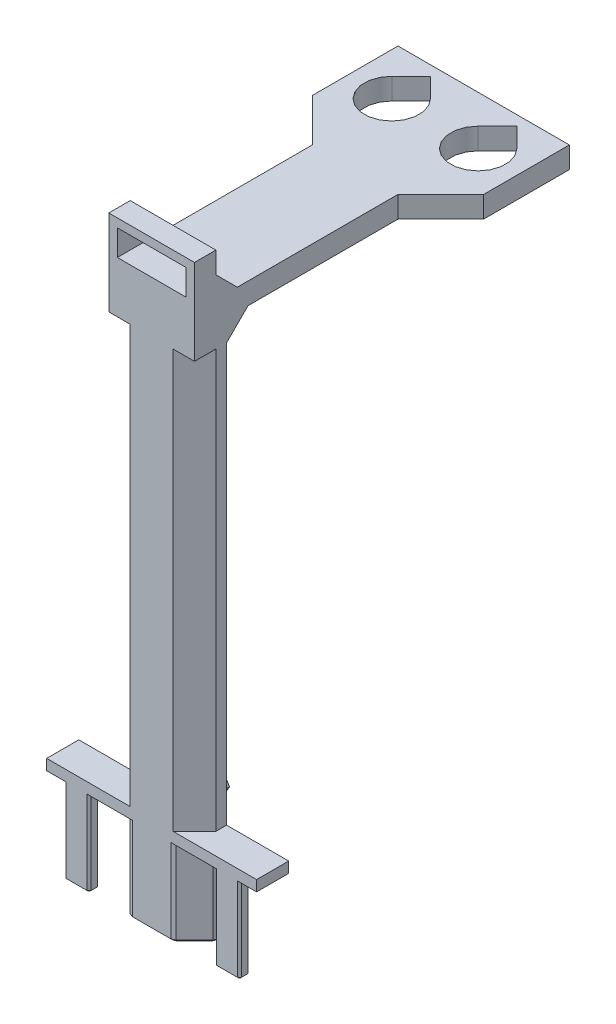
# Autodesk Inventor part: Vertical Beam Prototype
Saved by Autodesk Inventor 2022 (Build 260153000, 153)
## iProperties
Created: 2021-05-30
Part Number: Vertical Beam Prototype
Material: Generic
Document SubType Name: Modeling
Designer: sidsa
Density: 1 g/cm^3
Appearance: Silver
Author: sidsa
## iProperties of the stored document Vertical Beam Prototype_3DPrint.ipt
Created: 2021-05-30
Part Number: Vertical Beam Prototype_3DPrint
Material: Generic
Document SubType Name: Modeling
Designer: sidsa
Density: 1 g/cm^3
Appearance: Default
Author: sidsa
Autodesk Inventor part; units mm, degrees
ref_plane "YZ Plane" through (0, 0, 0) normal (1, 0, 0) x (0, 1, 0)
ref_plane "XZ Plane" through (0, 0, 0) normal (0, 1, 0) x (-1, 0, 0)
ref_plane "XY Plane" through (0, 0, 0) normal (0, 0, 1) x (1, 0, 0)
sketch "Sketch1" plane through (0, 0, 0) normal (0, 0, 1) x (1, 0, 0)
  line L0 (0, 0) -> (25.4, 0)
  line L1 (25.4, 0) -> (25.4, 165.1)
  line L2 (25.4, 165.1) -> (0, 165.1)
  line L3 (0, 165.1) -> (0, 0)
  line L4 (16.2837, 38.7604) -> (19.9133, 32.4739)
  line L5 (19.9133, 32.4739) -> (16.2837, 26.1874)
  line L6 (16.2837, 26.1874) -> (9.0247, 26.1874)
  line L7 (9.0247, 26.1874) -> (5.3952, 32.4739)
  line L8 (5.3952, 32.4739) -> (9.0247, 38.7604)
  line L9 (9.0247, 38.7604) -> (16.2837, 38.7604)
  line L10 (12.7, 0) -> (12.6542, 32.4739)
  dimension "d0" = 25.4
  dimension "d1" = 165.1
  dimension "d2" = 12.573
  dimension "d3" = 26.1874
  constraints: 22 end point, 3 parallel, 1 horizontal, 1 midpoint, 1 perpendicular, 13 other
  measures "d0" distance of L1.end L2.end
  measures "d1" distance of L0.end L1.end
  measures "d2" distance between parallel lines of L6 L9
  measures "d3" distance between parallel lines of L0 L6
extrude "Extrusion1" add sketch "Sketch1" along normal blind 3.175
sketch "Sketch2" plane through (0, 0, 0) normal (0, 0, -1) x (-1, 0, 0)
  line L0 (-25.4, 0) -> (-25.4, 165.1) projected
  line L1 (0, 0) -> (-25.4, 0) projected
  line L2 (0, 165.1) -> (0, 0) projected
  line L3 (-25.4, 165.1) -> (0, 165.1) projected
  line L4 (-16.2837, 26.1874) -> (-9.0247, 26.1874) projected
  line L5 (-19.9133, 32.4739) -> (-16.2837, 26.1874) projected
  line L6 (-16.2837, 38.7604) -> (-19.9133, 32.4739) projected
  line L7 (-9.0247, 38.7604) -> (-16.2837, 38.7604) projected
  line L8 (-5.3952, 32.4739) -> (-9.0247, 38.7604) projected
  line L9 (-9.0247, 26.1874) -> (-5.3952, 32.4739) projected
  line L10 (-16.2984, 26.1967) -> (-19.9179, 32.4658) projected
  line L11 (-5.4399, 32.4658) -> (-9.0594, 26.1967) projected
  line L12 (-9.0594, 26.1967) -> (-16.2984, 26.1967) projected
  line L13 (-16.2984, 26.1967) -> (-19.9179, 32.4658) projected
  line L14 (-19.9179, 32.4658) -> (-16.2984, 38.735) projected
  line L15 (-16.2984, 38.735) -> (-9.0594, 38.735) projected
  line L16 (-9.0594, 38.735) -> (-5.4399, 32.4658) projected
  line L17 (-41.2539, 1.27) -> (-34.9039, 1.27) projected
  line L18 (15.8961, 1.27) -> (15.8961, 63.5) projected
  line L19 (-41.2539, 63.5) -> (15.8961, 63.5) projected
  line L20 (-41.2539, 1.27) -> (-41.2539, 63.5) projected
  line L21 (6.3711, 1.27) -> (6.3711, 26.67) projected
  line L22 (6.3711, 26.67) -> (9.5461, 26.67) projected
  line L23 (9.5461, 26.67) -> (9.5461, 1.27) projected
  line L24 (9.5461, 1.27) -> (15.8961, 1.27) projected
  line L25 (-34.9039, 1.27) -> (-34.9039, 26.67) projected
  line L26 (-34.9039, 26.67) -> (-31.7289, 26.67) projected
  line L27 (-31.7289, 26.67) -> (-31.7289, 1.27) projected
  line L28 (-31.7289, 1.27) -> (6.3711, 1.27) projected
  dimension "d32" = 12.573
  dimension "d33" = 12.5383
  measures "d32" distance between parallel lines of L7 L4
  measures "d33" distance between parallel lines of L12 L15
extrude "Extrusion2" add sketch "Sketch2" along normal blind 6.35 and the other way blind 3.175 contours L5 L12 L11 L16 L15 L6 L7 L8 L9 L4 | L5 L6 L15 L16 L11 L12
sketch "Sketch3" plane through (0, 0, 3.175) normal (0, 0, 1) x (1, 0, 0)
  line L0 (25.4, 0) -> (25.4, 165.1) projected
  line L1 (25.4, 165.1) -> (0, 165.1) projected
  line L2 (0, 165.1) -> (0, 0) projected
  line L3 (0, 0) -> (25.4, 0) projected
extrude "Extrusion3" add sketch "Sketch3" along normal blind 6.35
chamfer "Chamfer1" distance 6.35 angle 45 2 edges at (25.4, 82.55, 9.525) (0, 82.55, 9.525)
sketch "Sketch5" plane through (9.0247, 38.7604, 0) normal (0, 1, 0) x (1, 0, 0)
  line L0 (7.259, 0) -> (7.259, 6.35) projected
  line L1 (32.2292, 2.54) -> (-24.9208, 2.54) projected
  line L2 (0, 0) -> (0, 6.35) projected
  line L3 (7.259, 0) -> (7.259, 6.35) projected
  line L4 (0, 6.35) -> (0, 0) projected
  line L5 (7.259, 2.54) -> (0, 2.54)
  line L6 (0, 2.54) -> (0, 6.35)
  line L7 (0, 6.35) -> (7.259, 6.35)
  line L8 (7.259, 6.35) -> (7.259, 2.54)
  line L9 (5.989, 3.175) -> (1.27, 3.175)
  line L10 (1.27, 3.175) -> (1.27, 5.715)
  line L11 (1.27, 5.715) -> (5.989, 5.715)
  line L12 (5.989, 5.715) -> (5.989, 3.175)
  point P0 (-9.0247, 0)
  dimension "d25" = 0.635
  dimension "d26" = 1.27
  dimension "d27" = 0.635
  dimension "d28" = 1.27
  dimension "d29" = 2.54
  constraints: 16 end point, 4 parallel, 2 horizontal, 2 perpendicular, 2 point on line
  measures "d25" distance between parallel lines of L1 L9
  measures "d26" distance between parallel lines of L2 L10
  measures "d27" distance between parallel lines of L7 L11
  measures "d28" distance between parallel lines of L0 L12
  measures "d29" distance between parallel lines of L11 L9
extrude "Extrusion5" cut sketch "Sketch5" against normal blind 12.7 contours L9 L10 L11 L12
sketch "Sketch6" plane through (0, 0, 0) normal (0, 0, -1) x (-1, 0, 0)
  line L0 (-25.4, 0) -> (-25.4, 165.1) projected
  line L1 (0, 0) -> (-25.4, 0) projected
  line L2 (0, 165.1) -> (0, 0) projected
  line L3 (-25.4, 165.1) -> (0, 165.1) projected
  line L4 (-16.2837, 26.1874) -> (-9.0247, 26.1874) projected
  line L5 (-19.9133, 32.4739) -> (-16.2837, 26.1874) projected
  line L6 (-16.2837, 38.7604) -> (-19.9133, 32.4739) projected
  line L7 (-9.0247, 38.7604) -> (-16.2837, 38.7604) projected
  line L8 (-5.3952, 32.4739) -> (-9.0247, 38.7604) projected
  line L9 (-9.0247, 26.1874) -> (-5.3952, 32.4739) projected
  line L10 (0, 165.1) -> (0, 0) projected
  line L11 (-25.4, 165.1) -> (0, 165.1)
  line L12 (0, 165.1) -> (0, 158.75)
  line L13 (0, 158.75) -> (-25.4, 158.75)
  line L14 (-25.4, 158.75) -> (-25.4, 165.1)
  point P0 (-25.4, 158.75)
  dimension "d34" = 6.35
  constraints: 8 end point, 2 parallel, 1 horizontal, 1 perpendicular, 1 point on line
  measures "d34" distance of L11.end L12.end
extrude "Extrusion6" add sketch "Sketch6" along normal blind 88.9 contours L0 L3 L2 L13
sketch "Sketch7" plane through (0, 0, 3.175) normal (-1, 0, 0) x (0, 0, 1)
  line L0 (-92.075, 165.1) -> (0, 165.1) projected
  line L1 (-3.175, 158.75) -> (-92.075, 158.75) projected
  line L2 (-92.075, 165.1) -> (-66.675, 165.1)
  line L3 (-66.675, 165.1) -> (-66.675, 158.75)
  line L4 (-66.675, 158.75) -> (-92.075, 158.75)
  line L5 (-92.075, 158.75) -> (-92.075, 165.1)
  point P0 (-3.175, 0)
  dimension "d37" = 25.4
  constraints: 8 end point, 2 parallel, 1 horizontal, 1 perpendicular, 1 point on line
  measures "d37" distance of L3.end L4.end
extrude "Extrusion7" add sketch "Sketch7" along normal blind 12.7
sketch "Sketch8" plane through (25.4, 0, 3.175) normal (1, 0, 0) x (0, 0, -1)
  line L0 (92.075, 165.1) -> (0, 165.1) projected
  line L1 (92.075, 165.1) -> (66.675, 165.1)
  line L2 (66.675, 165.1) -> (66.675, 158.75)
  line L3 (66.675, 158.75) -> (92.075, 158.75)
  line L4 (92.075, 158.75) -> (92.075, 165.1)
  point P0 (3.175, 0)
  dimension "d40" = 25.4
  dimension "d41" = 6.35
  constraints: 8 end point, 2 parallel, 1 horizontal, 1 perpendicular
  measures "d40" distance of L3.end L2.end
  measures "d41" distance of L2.end L1.end
extrude "Extrusion8" add sketch "Sketch8" along normal blind 12.7
sketch "Sketch9" plane through (6.35, 165.1, 9.525) normal (0, 1, 0) x (1, 0, 0)
  circle A0 centre (-6.227, 72.0756) radius 6.55 projected
  circle A1 centre (19.373, 72.0756) radius 6.55 projected
  line L0 (31.75, 98.425) -> (31.75, 73.025) projected
  line L1 (-19.05, 73.025) -> (-19.05, 98.425) projected
  line L2 (31.75, 73.025) -> (31.75, 98.425) projected
  line L3 (31.75, 83.986) -> (25.8752, 83.986)
  line L4 (12.8707, 83.986) -> (-19.05, 83.986)
  line L5 (31.75, 83.986) -> (27.2796, 83.986)
  line L6 (27.2796, 83.986) -> (19.1516, 83.986)
  circle A2 centre (19.1516, 83.986) radius 8.128
  line L7 (-19.05, 83.986) -> (-6.4516, 83.986)
  circle A3 centre (-6.4516, 83.986) radius 8.128
  line L8 (5.0431, 83.986) -> (-6.4516, 72.4913)
  line L9 (-6.4516, 72.4913) -> (-17.9463, 83.986)
  line L10 (-17.9463, 83.986) -> (-6.4516, 95.4808)
  line L11 (-6.4516, 95.4808) -> (5.0431, 83.986)
  line L12 (1.6764, 75.858) -> (-14.5796, 92.114) construction
  line L13 (-14.5796, 75.858) -> (1.6764, 92.114) construction
  line L14 (27.2796, 75.858) -> (11.0236, 75.858)
  line L15 (19.1516, 72.4913) -> (7.6569, 83.986)
  line L16 (7.6569, 83.986) -> (19.1516, 95.4808)
  line L17 (19.1516, 95.4808) -> (30.6463, 83.986)
  line L18 (27.2796, 75.858) -> (11.0236, 92.114) construction
  line L19 (11.0236, 75.858) -> (27.2796, 92.114) construction
  point P0 (-6.35, 9.525)
  point P1 (1.6764, 83.986)
  point P2 (-14.5796, 83.986)
  point P3 (-12.7293, 71.286)
  point P4 (0.2752, 71.286)
  point P5 (-2.0719, 77.1389)
  point P6 (-10.5701, 76.9787)
  point P7 (24.899, 89.7334)
  point P8 (13.4042, 89.7334)
  point P9 (-0.7042, 89.7334)
  point P10 (-12.199, 89.7334)
  dimension "d49" = 25.6
  dimension "d50" = 4.4704
  dimension "d51" = 8.128
  dimension "d52" = 16.256
  dimension "d53" = 12.5984
  dimension "d54" = 16.256
  constraints: 34 end point, 4 midpoint, 3 parallel, 3 perpendicular, 3 point on line, 2 centre point, 2 coincident, 1 horizontal
  measures "d49" distance of A0.centre A1.centre
  measures "d50" distance of L3.start L5.end
  measures "d51" distance of L5.end L6.end
  measures "d52" diameter of A2
  measures "d53" distance of L4.end L7.end
  measures "d54" diameter of A3
extrude "Extrusion9" cut sketch "Sketch9" against normal blind 6.35 contours A3 A0 | A0 A3 L4 | L4 A3 | A3 L10 L11 | A2 A1 | A1 A2 | A2 L16 L17
chamfer "Chamfer6" distance 6.35 angle 45 1 edges at (12.7, 158.75, 0)
sketch "Sketch10" plane through (0, 0, 3.175) normal (-1, 0, 0) x (0, 0, 1)
  line L0 (-9.525, 158.75) -> (-66.675, 158.75) projected
  line L1 (-3.175, 152.4) -> (-9.525, 158.75) projected
  line L2 (-3.175, 152.4) -> (-3.175, 0) projected
  line L3 (-3.175, 0) -> (0, 0) projected
  line L4 (0, 165.1) -> (0, 0) projected
  line L5 (-66.675, 165.1) -> (0, 165.1) projected
  line L6 (-9.525, 158.75) -> (-9.525, 165.1)
  line L7 (-3.175, 152.4) -> (6.35, 152.4)
  line L8 (6.35, 0) -> (6.35, 165.1) projected
  line L9 (6.35, 165.1) -> (-9.525, 165.1)
  line L10 (-66.675, 165.1) -> (-66.675, 158.75) projected
  constraints: 6 end point, 2 perpendicular, 2 point on line, 1 parallel
extrude "Extrusion10" add sketch "Sketch10" against normal blind 25.4 contours L6 L5 L4 L7 L1 | L4 L9 L8 L7
sketch "Sketch12" plane through (0, 0, 0) normal (0, -1, 0) x (1, 0, 0)
  line L0 (0, 3.175) -> (6.35, 9.525) projected
  line L1 (0, 0) -> (0, 3.175) projected
  line L2 (0, 0) -> (25.4, 0) projected
  line L3 (25.4, 0) -> (25.4, 3.175) projected
  line L4 (19.05, 9.525) -> (25.4, 3.175) projected
  line L5 (6.35, 9.525) -> (19.05, 9.525) projected
  line L6 (6.35, 9.525) -> (19.05, 9.525) projected
  line L7 (12.7, 9.525) -> (-18.415, 9.525)
  line L8 (12.7, 9.525) -> (43.815, 9.525)
  line L9 (43.815, 9.525) -> (43.815, 0)
  line L10 (43.815, 0) -> (-18.415, 0)
  line L11 (-18.415, 0) -> (-18.415, 9.525)
  dimension "d74" = 31.115
  dimension "d75" = 31.115
  constraints: 10 end point, 3 perpendicular, 2 point on line, 1 midpoint
  measures "d74" distance of L7.start L7.end
  measures "d75" distance of L7.start L8.end
extrude "Extrusion12" add sketch "Sketch12" against normal blind 3.175 contours L1 L10 L11 L7 L0 | L3 L4 L8 L9 L10
sketch "Sketch13" plane through (0, 3.175, 0) normal (0, 1, 0) x (1, 0, 0)
  line L0 (0, 0) -> (-18.415, 0) projected
  line L1 (-18.415, 0) -> (-18.415, -9.525) projected
  line L2 (-18.415, -9.525) -> (6.35, -9.525) projected
  line L3 (0, -3.175) -> (6.35, -9.525) projected
  line L4 (0, 0) -> (0, -3.175) projected
  line L5 (19.05, -9.525) -> (43.815, -9.525) projected
  line L6 (43.815, -9.525) -> (43.815, 0) projected
  line L7 (43.815, 0) -> (25.4, 0) projected
  line L8 (25.4, -3.175) -> (25.4, 0) projected
  line L9 (19.05, -9.525) -> (25.4, -3.175) projected
  line L10 (0, -9.525) -> (25.4, -9.525) projected
  line L11 (12.7, -9.525) -> (12.7, 5.0983)
  line L12 (9.0247, 6.35) -> (16.2837, 6.35) projected
  line L13 (43.815, -9.525) -> (-18.415, -9.525) projected
  line L14 (-13.335, -9.525) -> (-5.842, -9.525)
  line L15 (-5.842, -9.525) -> (-5.842, -6.35)
  line L16 (-5.842, -6.35) -> (-13.335, -6.35)
  line L17 (-13.335, -6.35) -> (-13.335, -9.525)
  line L18 (38.735, -9.525) -> (31.242, -9.525)
  line L19 (31.242, -9.525) -> (31.242, -6.35)
  line L20 (31.242, -6.35) -> (38.735, -6.35)
  line L21 (38.735, -6.35) -> (38.735, -9.525)
  point P0 (31.242, -9.525)
  dimension "d85" = 3.175
  dimension "d86" = 5.08
  dimension "d87" = 12.573
  constraints: 18 end point, 4 symmetric about line, 2 parallel, 2 perpendicular, 1 horizontal, 1 midpoint, 1 point on line
  measures "d85" distance between parallel lines of L13 L16
  measures "d86" distance between parallel lines of L1 L17
  measures "d87" distance between parallel lines of L1 L15
extrude "Extrusion13" add sketch "Sketch13" along normal blind 25.4 contours L17 L16 L15 L2 | L19 L20 L21 L5
fillet "Fillet1" radius 3.175 2 edges at (43.815, 1.5875, 9.525) (-18.415, 1.5875, 9.525)
sketch "Sketch14" plane through (0, 28.575, 0) normal (0, 1, 0) x (1, 0, 0)
  point P0 (0, 0)
sketch "Sketch15" plane through (0, 28.575, 0) normal (0, 1, 0) x (1, 0, 0)
  line L0 (0, 0) -> (-18.415, 0)
  line L1 (-18.415, 0) -> (-18.415, -9.525)
  line L2 (-18.415, -9.525) -> (6.35, -9.525)
  line L3 (0, -3.175) -> (6.35, -9.525)
  line L4 (0, 0) -> (0, -3.175)
  line L5 (19.05, -9.525) -> (43.815, -9.525)
  line L6 (43.815, -9.525) -> (43.815, 0)
  line L7 (43.815, 0) -> (25.4, 0)
  line L8 (25.4, -3.175) -> (25.4, 0)
  line L9 (19.05, -9.525) -> (25.4, -3.175)
  line L10 (0, -9.525) -> (25.4, -9.525)
  line L11 (12.7, -9.525) -> (12.7, 5.0983)
  line L12 (9.0247, 6.35) -> (16.2837, 6.35)
  line L13 (43.815, -9.525) -> (-18.415, -9.525)
  line L14 (-13.335, -9.525) -> (-5.715, -9.525)
  line L15 (-5.715, -9.525) -> (-5.715, -6.35)
  line L16 (-5.715, -6.35) -> (-13.335, -6.35)
  line L17 (-13.335, -6.35) -> (-13.335, -9.525)
  line L18 (38.735, -9.525) -> (31.115, -9.525)
  line L19 (31.115, -6.35) -> (38.735, -6.35)
  line L20 (38.735, -6.35) -> (38.735, -9.525)
  line L21 (31.115, -9.525) -> (31.115, -6.35)
  dimension "d91" = 3.175
  dimension "d92" = 5.08
  dimension "d93" = 12.7
  constraints: 44 end point, 4 symmetric about line, 2 parallel, 2 perpendicular, 1 horizontal, 1 midpoint, 1 point on line
  measures "d91" distance between parallel lines of L13 L16
  measures "d92" distance between parallel lines of L1 L17
  measures "d93" distance between parallel lines of L1 L15
extrude "Extrusion14" add sketch "Sketch15" against normal blind 3.175 contours L4 L3 L2 L15 L16 L17 L1 L0 | L9 L8 L7 L6 L5 L20 L19 L21
sketch "Sketch16" plane through (0, 3.175, 0) normal (0, 1, 0) x (1, 0, 0)
  arc A0 (-18.415, -6.35) -> (-15.24, -9.525) centre (-15.24, -6.35) ccw projected
  line L0 (-15.24, -9.525) -> (-13.335, -9.525) projected
  line L1 (-13.335, -9.525) -> (-13.335, -6.35) projected
  line L2 (-13.335, -6.35) -> (-5.842, -6.35) projected
  line L3 (-5.842, -6.35) -> (-5.842, -9.525) projected
  line L4 (-5.842, -9.525) -> (6.35, -9.525) projected
  line L5 (0, -3.175) -> (6.35, -9.525) projected
  line L6 (0, 0) -> (0, -3.175) projected
  line L7 (0, 0) -> (-18.415, 0) projected
  line L8 (-18.415, 0) -> (-18.415, -6.35) projected
  arc A1 (40.64, -9.525) -> (43.815, -6.35) centre (40.64, -6.35) ccw projected
  line L9 (43.815, -6.35) -> (43.815, 0) projected
  line L10 (43.815, 0) -> (25.4, 0) projected
  line L11 (25.4, -3.175) -> (25.4, 0) projected
  line L12 (19.05, -9.525) -> (25.4, -3.175) projected
  line L13 (19.05, -9.525) -> (31.242, -9.525) projected
  line L14 (31.242, -9.525) -> (31.242, -6.35) projected
  line L15 (31.242, -6.35) -> (38.735, -6.35) projected
  line L16 (38.735, -6.35) -> (38.735, -9.525) projected
  line L17 (38.735, -9.525) -> (40.64, -9.525) projected
extrude "Extrusion15" cut sketch "Sketch16" against normal blind 3.175
chamfer "Chamfer11" distance 0.635 angle 45 8 edges at (31.242, 12.7, 6.35) (31.242, 14.2875, 9.525) (38.735, 12.7, 9.525) (38.735, 12.7, 6.35) (-5.842, 12.7, 6.35) (-13.335, 12.7, 6.35) (-13.335, 12.7, 9.525) (-5.842, 14.2875, 9.525)
chamfer "Chamfer12" distance 0.635 angle 45 4 edges at (6.35, 12.7, 9.525) (0, 12.7, 3.175) (19.05, 12.7, 9.525) (25.4, 12.7, 3.175)
chamfer "Chamfer13" distance 0.635 angle 45 26 edges at (25.1755, 0, 3.082) (31.242, 0, 7.9375) (3.175, 0, 6.35) (12.7, 0, 0) (0, 0, 1.27) (0.2245, 0, 3.082) (12.7, 0, 9.525) (6.443, 0, 9.3005) (18.957, 0, 9.3005) (38.4175, 0, 6.6675) (34.9885, 0, 6.35) (22.225, 0, 6.35) (38.735, 0, 7.9375) (38.4175, 0, 9.2075) (34.9885, 0, 9.525) (31.5595, 0, 9.2075) (31.5595, 0, 6.6675) (25.4, 0, 1.27) (-13.335, 0, 7.9375) (-6.1595, 0, 6.6675) (-13.0175, 0, 9.2075) (-13.0175, 0, 6.6675) (-9.5885, 0, 9.525) (-9.5885, 0, 6.35) (-6.1595, 0, 9.2075) (-5.842, 0, 7.9375)
sketch "Sketch20" plane through (-12.7, 165.1, -88.9) normal (0, 1, 0) x (1, 0, 0)
  point P0 (12.7, -88.9)
sketch "Sketch21" plane through (0, 0, 9.525) normal (0, 0, 1) x (1, 0, 0)
  line L0 (-18.415, 28.575) -> (-18.415, 25.4) projected
  line L1 (43.815, 28.575) -> (43.815, 25.4) projected
  line L2 (-18.415, 28.575) -> (43.815, 28.575)
  line L3 (43.815, 28.575) -> (43.815, 25.4)
  line L4 (43.815, 25.4) -> (-18.415, 25.4)
  line L5 (-18.415, 25.4) -> (-18.415, 28.575)
  point P0 (0, 0)
  constraints: 8 end point, 2 parallel, 1 horizontal, 1 perpendicular
extrude "Extrusion18" add sketch "Sketch21" against normal blind 5.08
chamfer "Chamfer14" distance 12.7 angle 45 2 edges at (25.4, 161.925, -63.5) (0, 161.925, -63.5)
sketch "Sketch23" plane through (0, 0, 9.525) normal (0, 0, 1) x (1, 0, 0)
  line L0 (0, 152.4) -> (0, 165.1) projected
  line L1 (0, 165.1) -> (25.4, 165.1)
  line L2 (25.4, 165.1) -> (25.4, 177.8)
  line L3 (25.4, 177.8) -> (0, 177.8)
  line L4 (0, 177.8) -> (0, 165.1)
  line L5 (2.54, 175.26) -> (22.86, 175.26)
  line L6 (22.86, 175.26) -> (22.86, 167.64)
  line L7 (22.86, 167.64) -> (2.54, 167.64)
  line L8 (2.54, 167.64) -> (2.54, 175.26)
  point P0 (0, 0)
  dimension "d138" = 12.7
  dimension "d139" = 2.54
  constraints: 16 end point, 4 parallel, 2 perpendicular, 1 horizontal, 3 other
  measures "d138" distance of L1.end L2.end
  measures "d139" distance between parallel lines of L3 L5
extrude "Extrusion20" add sketch "Sketch23" against normal blind 6.35
chamfer "Chamfer17" distance 6.35 angle 45 1 edges at (12.7, 165.1, 3.175)
body "Solid1"
